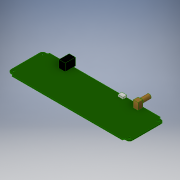
# Autodesk Inventor part: MainPCB
Saved by Autodesk Inventor 2017 (Build 210142000, 142)
## iProperties
Created: 2017-04-14
Part Number: MainPCB
Material: Generic
Document SubType Name: Sheet Metal
Designer: jeffkub
Density: 1 g/cm^3
Sheet Metal Rule: Default_mm
Appearance: Default(2)
Author: jeffkub
Autodesk Inventor part; units mm, degrees
ref_plane "YZ Plane" through (0, 0, 0) normal (1, 0, 0) x (0, 1, 0)
ref_plane "XZ Plane" through (0, 0, 0) normal (0, 1, 0) x (-1, 0, 0)
ref_plane "XY Plane" through (0, 0, 0) normal (0, 0, 1) x (1, 0, 0)
sketch "Sketch2" plane through (0, 0, 0) normal (0, 1, 0) x (-1, 0, 0)
  line L0 (101.6465, 0) -> (-102.4493, 0)
  line L1 (0, -49.7697) -> (0, 40.9396)
  line L2 (0, -27.5) -> (80, -27.5)
  line L3 (88, -27.5) -> (88, -25) construction
  line L4 (84, -25) -> (82, -25)
  line L5 (80.5, -26.5) -> (80.5, -27)
  line L6 (88, -21) -> (88, 0)
  line L7 (80.5, -27.5) -> (88, -27.5) construction
  arc A0 (84, -25) -> (88, -21) centre (84, -21) ccw
  arc A1 (82, -25) -> (80.5, -26.5) centre (82, -26.5) ccw
  arc A2 (80, -27.5) -> (80.5, -27) centre (80, -27) ccw
  circle A3 centre (84, -21) radius 1.6
  point P0 (0, 0)
  dimension "d7" = 176
  dimension "d8" = 55
  dimension "d9" = 2.5
  dimension "d10" = 7.5
  dimension "d11" = 4
  dimension "d12" = 1.5
  dimension "d13" = 0.5
  dimension "d16" = 3.2
  constraints: 16 end point, 8 point on line, 6 point on circle, 6 tangent, 4 centre point, 4 horizontal, 4 perpendicular, 1 coincident, 1 vertical
  measures "d7" diameter of L3 L1
  measures "d8" diameter of L2 L0
  measures "d9" distance between parallel lines of L4 L2
  measures "d10" distance between parallel lines of L5 L3
  measures "d11" radius of A0
  measures "d12" radius of A1
  measures "d13" radius of A2
  measures "d16" diameter of A3
extrude "Extrusion1" add sketch "Sketch2" along normal blind 1.6
mirror "Mirror1" about plane through (0, 0, 0) normal (0, 0, 1) of "Extrusion1"
mirror "Mirror2" about plane through (0, 0, 0) normal (1, 0, 0) of "Extrusion1", "Mirror1"
sketch "Sketch3" plane through (0, 1.6, 0) normal (0, 1, 0) x (1, 0, 0)
  line L0 (-54.5, 30) -> (-45.5, 30)
  line L1 (-45.5, 30) -> (-45.5, 15.2)
  line L2 (-45.5, 15.2) -> (-54.5, 15.2)
  line L3 (-54.5, 15.2) -> (-54.5, 30)
  point P0 (0, 0)
  point P1 (-50, 25)
  point P2 (-50, 30)
  dimension "d17" = 50
  dimension "d18" = 25
  dimension "d19" = 9
  dimension "d20" = 14.8
  dimension "d21" = 5
  constraints: 8 end point, 2 parallel, 1 horizontal, 1 midpoint, 1 perpendicular, 1 vertical alignment
  measures "d17" horizontal distance of point (0, 0) point (-50, 25)
  measures "d18" vertical distance of point (0, 0) point (-50, 25)
  measures "d19" distance of L0.start L0.end
  measures "d20" distance of L0.end L1.end
  measures "d21" distance from line of L0 point (-50, 25)
extrude "Extrusion2" add sketch "Sketch3" along normal blind 11
sketch "Sketch4" plane through (-45.5, 1.6, -30) normal (0, 0, -1) x (-1, 0, 0)
  circle A0 centre (4.5, 6.5) radius 3.25
  line L0 (0, 11) -> (9, 11) projected
  line L1 (9, 0) -> (0, 0) projected
  circle A1 centre (4.5, 6.5) radius 1
  point P0 (-45.5, -1.6)
  point P1 (4.5, 11)
  point P2 (4.5, 11)
  dimension "d24" = 6.5
  dimension "d25" = 6.5
  dimension "d26" = 2
  constraints: 2 centre point, 2 midpoint, 1 coincident, 1 vertical alignment
  measures "d24" distance from line of A0.centre L1
  measures "d25" diameter of A0
  measures "d26" diameter of A1
extrude "Extrusion3" cut sketch "Sketch4" against normal blind 11
sketch "Sketch5" plane through (0, 1.6, 0) normal (0, 1, 0) x (1, 0, 0)
  line L0 (56, 19.4) -> (49, 19.4)
  line L1 (49, 19.4) -> (49, 26.4)
  line L2 (49, 26.4) -> (56, 26.4)
  line L3 (56, 26.4) -> (56, 19.4)
  line L4 (56, 19.4) -> (49, 26.4) construction
  line L5 (49, 19.4) -> (56, 26.4) construction
  point P0 (0, 0)
  point P1 (52.5, 22.9)
  dimension "d29" = 52.5
  dimension "d30" = 22.9
  dimension "d31" = 7
  constraints: 12 end point, 2 midpoint, 2 parallel, 2 perpendicular, 1 horizontal
  measures "d29" horizontal distance of point (52.5, 22.9) point (0, 0)
  measures "d30" vertical distance of point (52.5, 22.9) point (0, 0)
  measures "d31" distance of L2.end L0.start
extrude "Extrusion4" add sketch "Sketch5" along normal blind 10
sketch "Sketch6" plane through (56, 1.6, -26.4) normal (0, 0, -1) x (-1, 0, 0)
  line L0 (0, 10) -> (7, 10) projected
  circle A0 centre (3.5, 6.6) radius 3.4
  line L1 (101.5, 0) -> (-24, 0) projected
  point P0 (56, -1.6)
  point P1 (3.5, 10)
  dimension "d34" = 6.6
  dimension "d35" = 6.8
  constraints: 1 centre point, 1 midpoint, 1 vertical alignment
  measures "d34" distance from line of A0.centre L1
  measures "d35" diameter of A0
extrude "Extrusion5" add sketch "Sketch6" along normal blind 1.1
sketch "Sketch7" plane through (52.5, 8.2, -27.5) normal (0, 0, -1) x (-1, 0, 0)
  circle A0 centre (0, 0) radius 3.4 projected
  circle A1 centre (0, 0) radius 3.175
  point P0 (52.5, -8.2)
  dimension "d38" = 6.35
  constraints: 1 centre point, 1 coincident
  measures "d38" diameter of A1
extrude "Extrusion6" add sketch "Sketch7" along normal blind 11.4 contours A1
sketch "Sketch8" plane through (0, 1.6, 0) normal (0, 1, 0) x (1, 0, 0)
  line L0 (23.75, 28.02) -> (31.25, 28.02)
  line L1 (31.25, 28.02) -> (31.25, 22.45)
  line L2 (31.25, 22.45) -> (23.75, 22.45)
  line L3 (23.75, 22.45) -> (23.75, 28.02)
  point P0 (0, 0)
  point P1 (27.5, 27.5)
  point P2 (27.5, 28.02)
  dimension "d41" = 27.5
  dimension "d42" = 27.5
  dimension "d43" = 5.05
  dimension "d44" = 0.52
  dimension "d45" = 7.5
  constraints: 8 end point, 2 parallel, 1 horizontal, 1 midpoint, 1 perpendicular, 1 vertical alignment
  measures "d41" horizontal distance of point (27.5, 27.5) point (0, 0)
  measures "d42" horizontal distance of point (27.5, 27.5) point (0, 0)
  measures "d43" distance from line of L2 point (27.5, 27.5)
  measures "d44" distance from line of L0 point (27.5, 27.5)
  measures "d45" distance of L1.end L2.end
extrude "Extrusion7" add sketch "Sketch8" along normal blind 2.7
equation "\"BendRadius\" = Thickness"
equation "\"BendReliefWidth\" = Thickness"
equation "\"BendReliefDepth\" = 0.5 * Thickness"
equation "\"CornerReliefSize\" = 4 * Thickness"
equation "\"MinimumRemnant\" = 2 * Thickness"
equation "\"TransitionRadius\" = BendRadius"
equation "\"JacobiRadiusSize\" = BendRadius"
equation "\"GapSize\" = Thickness"
equation "\"Thickness\" = 0.5"
body "Solid1"
